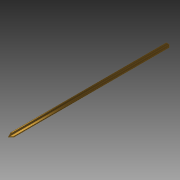
# Autodesk Inventor part: 2222_Brass Angle Bracket_V1
Saved by Autodesk Inventor 2020 (Build 240168000, 168)
## iProperties
Created: 2017-08-01
Part Number: 2222_Brass Angle Bracket_V1
Material: Brass
Document SubType Name: Modeling
Designer: MPI
Density: 8.49 g/cm^3
Appearance: Brass - Polished
Author: MPI
Autodesk Inventor part; units mm, degrees
ref_plane "YZ Plane" through (0, 0, 0) normal (1, 0, 0) x (0, 1, 0)
ref_plane "XZ Plane" through (0, 0, 0) normal (0, 1, 0) x (-1, 0, 0)
sketch "Sketch1" plane through (0, 0, 0) normal (0, 0, 1) x (1, 0, 0)
  line L0 (-5.3558, -5.3558) -> (5.3558, -5.3558)
  line L1 (5.3558, -5.3558) -> (5.3558, 5.3558)
  line L2 (5.3558, 5.3558) -> (-5.3558, 5.3558)
  line L3 (-5.3558, 5.3558) -> (-5.3558, -5.3558)
  line L4 (-5.3558, -5.3558) -> (5.3558, 5.3558) construction
  line L5 (5.3558, -5.3558) -> (-5.3558, 5.3558) construction
  line L6 (5.3558, 5.3558) -> (-2.1808, 5.3558)
  line L7 (-2.1808, 5.3558) -> (-2.1808, -2.1808)
  line L8 (-2.1808, -2.1808) -> (5.3558, -2.1808)
  line L9 (5.3558, -2.1808) -> (5.3558, 5.3558)
  point P0 (0, 0)
  dimension "d0" = 3.175
  dimension "d1" = 3.175
  constraints: 20 end point, 4 parallel, 2 horizontal, 2 midpoint, 2 perpendicular, 1 point on line
  measures "d0" distance between parallel lines of L0 L8
  measures "d1" distance between parallel lines of L3 L7
extrude "Extrusion1" add sketch "Sketch1" along normal blind 618.0836 contours L3 L2 L7 L8 L1 L0
sketch "Sketch2" plane through (-5.3558, -5.3558, 0) normal (-1, 0, 0) x (0, 0, 1)
  line L0 (0, 10.7115) -> (0, 0) projected
  line L1 (0, 0) -> (618.0836, 0) projected
  line L2 (0, 10.7115) -> (618.0836, 10.7115) projected
  line L3 (309.0418, 10.7115) -> (309.0418, 0)
  line L4 (618.0836, 0) -> (607.3721, 10.7115)
  line L5 (618.0836, 0) -> (633.232, 0) construction
  line L6 (607.3721, 10.7115) -> (618.0836, 10.7115)
  line L7 (618.0836, 0) -> (618.0836, 10.7115)
  line L8 (0, 10.7115) -> (0, 0)
  line L9 (0, 0) -> (10.7115, 10.7115)
  line L10 (0, 0) -> (-15.1484, 0) construction
  line L11 (10.7115, 10.7115) -> (0, 10.7115)
  line L12 (0, 0) -> (0, 10.7115)
  point P0 (0, 5.3558)
  dimension "d4" = 135
  constraints: 20 end point, 2 midpoint, 2 symmetric about line, 1 collinear, 1 equal length, 1 horizontal, 1 perpendicular, 1 point on line
  measures "d4" angle of L5 L4
extrude "Extrusion2" cut sketch "Sketch2" against normal blind 25.4 contours L2 L9 L0 | L4 L2 L7
ref_plane "Work Plane1" through (-2.1808, -2.1808, 614.9086) normal (-0.7071068, 0.7071068, 0) x (0, 0, 1)
mirror "Mirror1" about plane through (-2.1808, -2.1808, 614.9086) normal (-0.7071068, 0.7071068, 0) of "Extrusion2"
body "Solid1"
